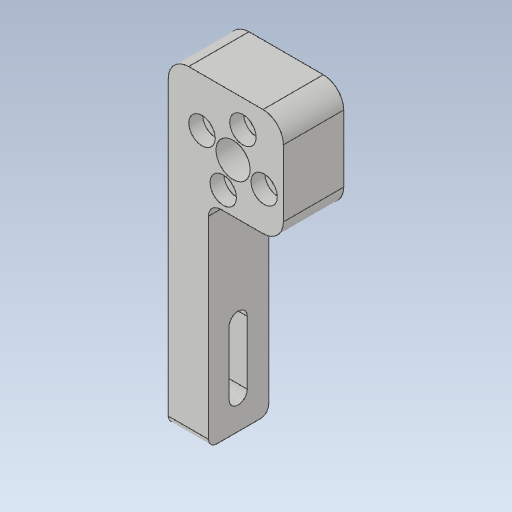
# Autodesk Inventor part: ZnutBracket
Saved by Autodesk Inventor 2020 (Build 240168000, 168)
## iProperties
Created: 2018-10-03
Part Number: ZnutBracket
Material: Generic
Document SubType Name: Modeling
Designer: LillaHunden
Density: 1 g/cm^3
Appearance: Default
Mass: 15.4031 g
Surface Area: 68.167 cm^2
Volume: 15.4031 cm^3
Author: LillaHunden
Autodesk Inventor part; units mm, degrees
ref_plane "Work Plane1" through (-20, -38.5, -25) normal (-1, 0, 0) x (0, 0, 1)
sketch "Sketch1" plane through (0, 0, 0) normal (0, 0, 1) x (1, 0, 0)
  line L0 (-7.75, 8.6987) -> (-7.75, 35.0829)
  line L1 (-7.75, 35.0829) -> (-36, 35.0829)
  line L2 (-36, 35.0829) -> (-36, -43.6977)
  line L3 (-36, -43.6977) -> (-20.05, -43.6977)
  line L4 (-20.05, -43.6977) -> (-20.05, -7.832)
  line L5 (-20.05, -7.832) -> (-26, -7.832)
  line L6 (-26, -7.832) -> (-26, 8.6987)
  line L7 (-26, 8.6987) -> (-7.75, 8.6987)
  line L8 (6.0684, -6.4305) -> (5.9986, -8.4293) construction
  line L9 (5.9986, -8.4293) -> (24.987, -9.0929) construction
  line L10 (24.987, -9.0929) -> (25.5109, 5.898) construction
  line L11 (25.5109, 5.898) -> (7.0721, 6.5424) construction
  line L12 (7.0721, 6.5424) -> (6.8975, 1.5454) construction
  line L13 (6.8975, 1.5454) -> (-6.1945, 2.0029) construction
  line L14 (-6.1945, 2.0029) -> (-6.0199, 6.9999) construction
  line L15 (-6.0199, 6.9999) -> (-24.4586, 7.6443) construction
  line L16 (-24.4586, 7.6443) -> (-24.9825, -7.3466) construction
  line L17 (-24.9825, -7.3466) -> (-5.9941, -8.0102) construction
  line L18 (-5.9941, -8.0102) -> (-5.9243, -6.0114) construction
  line L19 (-5.9243, -6.0114) -> (6.0684, -6.4305) construction
  line L20 (-6.0946, 1.9994) -> (-4.9312, 35.289) construction
  line L21 (6.8975, 1.5454) -> (-6.0946, 1.9994) construction
  line L22 (6.8975, 1.5454) -> (8.0609, 34.835) construction
  line L23 (19.6058, -19.9115) -> (-20.3698, -18.5145) construction
  line L24 (-20.3698, -18.5145) -> (-20.6492, -26.5096) construction
  line L25 (19.3264, -27.9067) -> (-20.6492, -26.5096) construction
  line L26 (19.6058, -19.9115) -> (19.3264, -27.9067) construction
  line L27 (296.5, -28.5) -> (282.6818, -28.5) construction
  line L28 (296.5, -38.5) -> (282.6818, -38.5) construction
  circle A0 centre (15.255, -1.2482) radius 1.621 projected
  circle A1 centre (-14.7267, -0.2004) radius 1.621 projected
  circle A2 centre (0.3032, 27.2914) radius 1.621 projected
  circle A3 centre (-0.3954, 7.3036) radius 1.621 projected
  line L29 (282.6818, -38.5) -> (282.6818, -28.5) projected
  line L30 (296.5, -28.5) -> (296.5, -38.5) projected
  line L31 (8.0609, 34.835) -> (-4.9312, 35.289) projected
  point P0 (0, 0)
  dimension "d8" = 10
  constraints: 16 end point, 7 perpendicular, 1 vertical, 1 other
  measures "d8" distance between parallel lines of L6 L2
extrude "Extrusion1" add sketch "Sketch1" along normal blind 14.8 contours L7 L6 L5 L4 L3 L2 L1 L0
sketch "Sketch2" plane through (0, 0, 14.8) normal (0, 0, 1) x (1, 0, 0)
  circle A0 centre (-20.1, 20.7) radius 5.15 construction
  circle A1 centre (-20.1, 20.7) radius 4.2
  point P0 (0, 0)
  dimension "d18" = 8.4
  constraints: 1 centre point
  measures "d18" diameter of A1
extrude "Extrusion2" cut sketch "Sketch2" against normal through all
sketch "Sketch8" plane through (-36, 35.0829, 0) normal (-1, 0, 0) x (0, 0, 1)
  circle A0 centre (32.5096, -69.8259) radius 2.5 construction
  circle A1 centre (32.5096, -69.8259) radius 3.5
  point P0 (0, -35.0829)
  dimension "d28" = 7
  constraints: 1 centre point, 1 coincident
  measures "d28" diameter of A1
sketch "Sketch9" plane through (-36, 35.0829, 0) normal (-1, 0, 0) x (0, 0, 1)
  circle A0 centre (32.5096, -69.8259) radius 3.5 projected
  circle A1 centre (32.5096, -69.8259) radius 10
  point P0 (0, -35.0829)
  dimension "d31" = 20
  constraints: 1 centre point, 1 coincident
  measures "d31" diameter of A1
sketch "Sketch10" plane through (-36, 35.0829, 0) normal (-1, 0, 0) x (0, 0, 1)
  line L0 (45.4011, -39.3798) -> (15, -39.3798) projected
  line L1 (45.4011, -39.3798) -> (104.8234, -39.3798)
  line L2 (104.8234, -39.3798) -> (104.8234, -112.1071)
  line L3 (104.8234, -112.1071) -> (45.4011, -112.1071)
  line L4 (45.4011, -112.1071) -> (45.4011, -39.3798)
  line L5 (0, 0) -> (0, -81.2089) projected
  line L6 (0, -81.2089) -> (45.4011, -81.2089)
  line L7 (45.4011, -81.2089) -> (45.4011, -112.1071)
  line L8 (45.4011, -112.1071) -> (0, -112.1071)
  line L9 (0, -112.1071) -> (0, -81.2089)
  point P0 (0, -35.0829)
  constraints: 16 end point, 4 parallel, 2 horizontal, 2 perpendicular
sketch "Sketch11" plane through (-36, 35.0829, 0) normal (-1, 0, 0) x (0, 0, 1)
  circle A0 centre (96.9549, -98.5564) radius 2.5 construction
  circle A1 centre (96.9549, -51.4164) radius 2.75 construction
  circle A2 centre (49.8149, -98.5564) radius 2.5 construction
  circle A3 centre (49.8149, -51.4164) radius 2.75 construction
  circle A4 centre (96.9549, -98.5564) radius 2.75 construction
  circle A5 centre (96.9549, -51.4164) radius 2.5 construction
  point P0 (0, -35.0829)
sketch "Sketch12" plane through (-20.05, -7.832, 15) normal (1, 0, 0) x (0, 0, -1)
  line L0 (-86.5849, -8.3715) -> (-86.5849, -44.0215) construction
  line L1 (-30.1849, -55.7715) -> (-30.1849, -20.1215) construction
  arc A0 (-34.6849, -60.2715) -> (-30.1849, -55.7715) centre (-34.6849, -55.7715) ccw construction
  line L2 (-39.1849, -60.2715) -> (-34.6849, -60.2715) construction
  arc A1 (-30.4349, -8.3715) -> (-34.6849, -4.1215) centre (-34.6849, -8.3715) ccw construction
  line L3 (-30.4349, -8.3715) -> (-30.4349, -12.6215) construction
  line L4 (-30.4349, -12.6215) -> (-33.6849, -12.6215) construction
  arc A2 (-33.6849, -12.6215) -> (-33.6849, -20.1215) centre (-33.6849, -16.3715) ccw construction
  line L5 (-33.6849, -20.1215) -> (-30.4349, -20.1215) construction
  line L6 (-30.4349, -20.1215) -> (-30.4349, -55.7715) construction
  arc A3 (-34.6849, -60.0215) -> (-30.4349, -55.7715) centre (-34.6849, -55.7715) ccw construction
  line L7 (-34.6849, -60.0215) -> (-38.9349, -60.0215) construction
  line L8 (-38.9349, -60.0215) -> (-38.9349, -56.7715) construction
  arc A4 (-38.9349, -56.7715) -> (-46.4349, -56.7715) centre (-42.6849, -56.7715) ccw construction
  line L9 (-46.4349, -56.7715) -> (-46.4349, -60.0215) construction
  line L10 (-46.4349, -60.0215) -> (-82.0849, -60.0215) construction
  arc A5 (-86.3349, -55.7715) -> (-82.0849, -60.0215) centre (-82.0849, -55.7715) ccw construction
  line L11 (-86.3349, -55.7715) -> (-86.3349, -51.5215) construction
  line L12 (-86.3349, -51.5215) -> (-83.0849, -51.5215) construction
  arc A6 (-83.0849, -51.5215) -> (-83.0849, -44.0215) centre (-83.0849, -47.7715) ccw construction
  line L13 (-83.0849, -44.0215) -> (-86.3349, -44.0215) construction
  line L14 (-86.3349, -44.0215) -> (-86.3349, -8.3715) construction
  arc A7 (-82.0849, -4.1215) -> (-86.3349, -8.3715) centre (-82.0849, -8.3715) ccw construction
  line L15 (-82.0849, -4.1215) -> (-77.8349, -4.1215) construction
  line L16 (-77.8349, -4.1215) -> (-77.8349, -7.3715) construction
  arc A8 (-77.8349, -7.3715) -> (-70.3349, -7.3715) centre (-74.0849, -7.3715) ccw construction
  line L17 (-70.3349, -7.3715) -> (-70.3349, -4.1215) construction
  line L18 (-70.3349, -4.1215) -> (-34.6849, -4.1215) construction
  circle A9 centre (-81.9549, -55.6415) radius 2.75 construction
  circle A10 centre (-81.9549, -8.5015) radius 2.75 construction
  circle A11 centre (-34.8149, -8.5015) radius 2.75 construction
  circle A12 centre (-34.8149, -55.6415) radius 2.75 construction
  circle A13 centre (-58.3849, -32.0715) radius 19.3 construction
  line L19 (-89.8234, -69.1922) -> (-89.8234, 3.5351) projected
  line L20 (-89.8234, 3.5351) -> (0, 3.5351) projected
  line L21 (-89.8234, -69.1922) -> (-26.5432, -69.1922)
  line L22 (-26.5432, -69.1922) -> (-26.5432, 3.5351)
  line L23 (-26.5432, 3.5351) -> (-89.8234, 3.5351)
  line L24 (-89.8234, 3.5351) -> (-89.8234, -69.1922)
  point P0 (15, 7.832)
  constraints: 8 end point, 2 parallel, 1 horizontal, 1 perpendicular, 1 point on line
sketch "Sketch13" plane through (-20.05, -7.832, 15) normal (0, 0, -1) x (-1, 0, 0)
  line L0 (0, 0) -> (5.25, 0) projected
  line L1 (5.25, 0) -> (5.25, 3.5351) projected
  line L2 (5.25, 3.5351) -> (0, 3.5351) projected
  line L3 (0, 3.5351) -> (0, 0) projected
  point P0 (-20.05, 7.832)
sketch "Sketch14" plane through (-35.3, -77.0243, 104.8234) normal (0, 0, 1) x (1, 0, 0)
  line L0 (15.25, 69.1922) -> (10, 69.1922) projected
  line L1 (10, 69.1922) -> (15.25, 69.1922)
  line L2 (15.25, 69.1922) -> (15.25, 0)
  line L3 (15.25, 0) -> (10, 0)
  line L4 (10, 0) -> (10, 69.1922)
  point P0 (35.3, 77.0243)
  constraints: 8 end point, 2 parallel, 1 horizontal, 1 perpendicular
sketch "Sketch15" plane through (-30.05, -7.832, 15) normal (1, 0, 0) x (0, 0, -1)
  circle A0 centre (-58.3849, -32.0715) radius 19.3 construction
  circle A1 centre (-58.3849, -32.0715) radius 20.384
  point P0 (15, 7.832)
  constraints: 1 centre point
sketch "Sketch16" plane through (-31.05, -39.9036, 73.3849) normal (1, 0, 0) x (0, 0, -1)
  circle A0 centre (0, 0) radius 2.675 construction
  circle A1 centre (0, 0) radius 3.5
  point P0 (73.3849, 39.9036)
  dimension "d51" = 7
  constraints: 1 centre point, 1 coincident
  measures "d51" diameter of A1
sketch "Sketch6" plane through (0, 0, 14.8) normal (0, 0, 1) x (1, 0, 0)
  point P0 (-17.6836, 28.3263)
  point P1 (-12.4737, 18.2836)
  point P2 (-22.5164, 13.0737)
  point P3 (-27.7263, 23.1164)
hole "Hole3" at (-17.6836, 28.3263, 14.8) at (-12.4737, 18.2836, 14.8) at (-22.5164, 13.0737, 14.8) at (-27.7263, 23.1164, 14.8) direction (0, 0, -1) diameter 3.4 depth 14.8 counterbore diameter 6.5 counterbore depth 3.4
sketch "Sketch17" plane through (0, 0, 14.8) normal (0, 0, 1) x (1, 0, 0)
  line L0 (-36, -43.6977) -> (-20.05, -43.6977) projected
  line L1 (-20.05, -43.6977) -> (-20.05, -7.832) projected
  line L2 (-26.1554, -43.6977) -> (-20.05, -43.6977)
  line L3 (-20.05, -43.6977) -> (-20.05, 8.6987)
  line L4 (-20.05, 8.6987) -> (-26.1554, 8.6987)
  line L5 (-26.1554, 8.6987) -> (-26.1554, -43.6977)
  point P0 (0, 0)
  point P1 (-26, 8.6987)
  constraints: 8 end point, 3 point on line, 2 parallel, 1 horizontal, 1 perpendicular
extrude "Extrusion12" cut sketch "Sketch17" against normal through all
fillet "Fillet1" radius 5 2 edges at (-36, 35.0829, 7.4) (-7.75, 35.0829, 7.4)
fillet "Fillet2" radius 5 1 edges at (-7.75, 8.6987, 7.4)
fillet "Fillet3" radius 3 1 edges at (-26.1554, 8.6987, 7.4)
fillet "Fillet4" radius 2 2 edges at (-31.0777, -43.6977, 0) (-31.0777, -43.6977, 14.8)
ref_plane "Work Plane2" through (0, 0, 7.4) normal (0, 0, -1) x (-1, 0, 0)
sketch "Sketch18" plane through (-36, 30.0829, 0) normal (-1, 0, 0) x (0, 0, 1)
  point P0 (7.5, -52.6646)
  point P1 (7.5, -63.6646)
  point P2 (-8.5, -52.6646)
  point P3 (-24.5, -52.6646)
  point P4 (47.5, -52.6646)
hole "Hole6" at (-36, -22.5817, 7.5) at (-36, -33.5817, 7.5) at (-36, -22.5817, -8.5) at (-36, -22.5817, -24.5) at (-36, -22.5817, 47.5) direction (1, 0, 0) diameter 4.5 depth 9.8446 counterbore diameter 8 counterbore depth 4.6
sketch "Sketch19" plane through (-36, 30.0829, 0) normal (-1, 0, 0) x (0, 0, 1)
  circle A0 centre (7.5, -52.6646) radius 4 projected
  circle A1 centre (7.5, -63.6646) radius 4 projected
  line L0 (7.5, -50.3269) -> (7.5, -65.9146) construction
  circle A2 centre (7.5, -63.6646) radius 2.25 projected
  line L1 (3.1638, -50.3269) -> (3.1638, -65.9146)
  line L2 (11.8362, -65.9146) -> (11.8362, -50.3269)
  arc A3 (11.8362, -50.3269) -> (3.1638, -50.3269) centre (7.5, -50.3269) ccw
  arc A4 (3.1638, -65.9146) -> (11.8362, -65.9146) centre (7.5, -65.9146) ccw
  point P0 (0, -30.0829)
  point P1 (7.5, -58.1207)
  constraints: 8 end point, 4 point on circle, 4 tangent, 2 centre point, 1 midpoint, 1 parallel, 1 vertical, 1 vertical alignment, 1 other
ref_plane "Work Plane3" through (-31.4, -26.0817, 4) normal (1, 0, 0) x (0, 1, 0)
extrude "Extrusion13" cut sketch "Sketch19" against normal up to surface (4.6 mm away) contours A3 L2 A4 L1
sketch "Sketch20" plane through (-31.4, -35.8317, 11.8362) normal (-1, 0, 0) x (0, 0, 1)
  circle A0 centre (-4.3362, 13.25) radius 2.25 projected
  line L0 (-4.3362, 15.5) -> (-4.3362, 0) construction
  circle A1 centre (-4.3362, 2.25) radius 2.25 projected
  line L1 (-2.0862, 15.5) -> (-2.0862, 0)
  line L2 (-6.5862, 0) -> (-6.5862, 15.5)
  arc A2 (-2.0862, 15.5) -> (-6.5862, 15.5) centre (-4.3362, 15.5) ccw
  arc A3 (-6.5862, 0) -> (-2.0862, 0) centre (-4.3362, 0) ccw
  point P0 (-11.8362, 35.8317)
  point P1 (-4.3362, 7.75)
  constraints: 8 end point, 4 point on circle, 4 tangent, 2 centre point, 2 vertical alignment, 1 midpoint, 1 parallel, 1 vertical, 2 other
extrude "Extrusion14" cut sketch "Sketch20" against normal through all contours L1 A1 L2 A0 | A0 L2 A2 L1 | L1 A3 L2 A1
chamfer "Chamfer1" distance 0.5 angle 45 4 edges at (-36, -28.0378, 11.8362) (-36, -40.1679, 7.5) (-36, -28.0378, 3.1638) (-36, -15.9078, 7.5)
body "Solid1"
